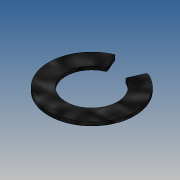
# Autodesk Inventor part: Circlip
Saved by Autodesk Inventor 2015 (Build 190159000, 159)
## iProperties
Created: 2016-12-08
Part Number: Circlip
Material: Allgemein
Document SubType Name: Modeling
Designer: NS
Density: 1 g/cm^3
Appearance: Black Cast
RuleStatus: InUse
BeforeDocSave0: file://C:\_Vault_ausgecheckt\ilogic\ipt
Author: NS
Autodesk Inventor part; units mm, degrees
ref_plane "YZ Plane" through (0, 0, 0) normal (1, 0, 0) x (0, 1, 0)
ref_plane "XZ Plane" through (0, 0, 0) normal (0, 1, 0) x (-1, 0, 0)
ref_plane "XY Plane" through (0, 0, 0) normal (0, 0, 1) x (1, 0, 0)
sketch "Sketch1" plane through (0, 0, 0) normal (0, 0, 1) x (1, 0, 0)
  arc A0 (-0.6137, 1.3687) -> (0.6137, 1.3687) centre (0, 0) ccw
  arc A1 (-1.013, 2.2856) -> (1.013, 2.2856) centre (0, 0) ccw
  line L0 (-0.8807, 2.2339) -> (-0.5628, 1.4997)
  line L1 (0.8807, 2.2339) -> (0.5628, 1.4997)
  arc A2 (-0.8807, 2.2339) -> (-1.013, 2.2856) centre (-0.9724, 2.1942) ccw
  arc A3 (-0.6137, 1.3687) -> (-0.5628, 1.4997) centre (-0.6546, 1.46) ccw
  arc A4 (0.5628, 1.4997) -> (0.6137, 1.3687) centre (0.6546, 1.46) ccw
  arc A5 (1.013, 2.2856) -> (0.8807, 2.2339) centre (0.9724, 2.1942) ccw
  point P0 (-0.5223, 1.4061)
  point P1 (0.5223, 1.4061)
  point P2 (-0.9199, 2.3246)
  point P3 (0.9199, 2.3246)
  point P4 (-0.9199, 2.3246)
  dimension "d0" = 1.5
  dimension "d1" = 2.5
  dimension "d2" = 0.1
  constraints: 17 point on circle, 8 tangent, 6 centre point, 4 end point, 4 point on line, 3 equal radius, 2 coincident, 2 horizontal alignment
  measures "d0" radius of A0
  measures "d1" radius of A1
  measures "d2" radius of A2
extrude "Extrusion1" add sketch "Sketch1" along normal blind 0.2
body "Solid1"
